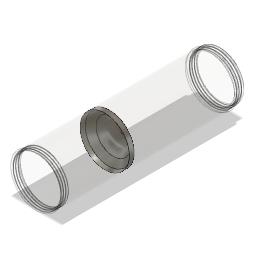
FalconHeavy-SideBoosterBase(No Fin) (Autodesk Fusion 360 design; units mm, degrees)
Autodesk Fusion 360 part; units mm, degrees
sketch "Sketch1" plane through (0, 0, 0) normal (0, 1, 0) x (1, 0, 0)
  line L0 (0, 0) -> (21, 0)
  line L1 (0, 0) -> (20.2, 0)
  line L2 (21, 0) -> (21, 144)
  line L3 (20.2, 0) -> (20.2, 144)
  line L4 (20.2, 144) -> (18.2, 144)
  line L5 (18.2, 144) -> (18.2, 150)
  line L6 (18.2, 150) -> (20.2, 150)
  line L7 (20.2, 150) -> (20.2, 144)
  line L8 (21, 144) -> (20.2, 144)
  line L9 (20.2, 144) -> (20.2, 142)
  spline S0 degree 5 poles (20.2, 142) (20.2, 142.0899) (20.1718, 142.2773) (20.045, 142.5812) (19.7343, 143.0169) (19.2169, 143.5343) (18.7812, 143.845) (18.4773, 143.9718) (18.2899, 144) (18.2, 144) knots 0 0 0 0 0 0 0.2 0.4 0.6 0.8 1 1 1 1 1 1
  line L10 (20.2, 141.8) -> (20.2, 142.2)
  line L11 (18.4, 144) -> (18, 144)
  line L12 (0, 0) -> (0, 150) construction
  line L13 (20.2, 0) -> (20.2, 6)
  line L14 (20.2, 6) -> (0, 6)
  line L15 (20.2, 6) -> (20.2, 7)
  line L16 (20.2, 7) -> (0, 7)
  line L17 (0, 7) -> (0, 6)
  dimension "d1" = 21
  dimension "d2" = 20.2
  dimension "d3" = 144
  dimension "d4" = 144
  dimension "d5" = 2
  dimension "d6" = 6
  dimension "d7" = 2
  dimension "d8" = 2
  dimension "d9" = 150
  dimension "d10" = 6
  dimension "d11" = 1
  constraint coincident L0.start L1.start
  constraint horizontal L0
  constraint parallel L0 L1
  constraint perpendicular L0 L2
  constraint perpendicular L1 L3
  constraint perpendicular L3 L4
  constraint perpendicular L4 L5
  constraint perpendicular L5 L6
  constraint perpendicular L4 L9
  constraint midpoint L9.end L10
  constraint coincident L3 L10.start
  constraint midpoint L4.end L11
  constraint perpendicular L0 L12
  constraint perpendicular L1 L13
  constraint perpendicular L3 L14
  constraint coincident L3 L15.end
  constraint coincident L12 L16.end
  constraint perpendicular L12 L16
  constraint perpendicular L14 L17
  measures "d1" distance of L0.start L0.end
  measures "d2" distance of L0.start L1.end
  measures "d3" distance of L0.end L2.end
  measures "d4" distance of L1.end L3.end
  measures "d5" distance of L3.end L4.end
  measures "d6" distance of L4.end L5.end
  measures "d7" distance of L5.end L6.end
  measures "d8" distance of L3.end L9.end
  measures "d9" distance of L0.start L12.end
  measures "d10" distance of L1.end L13.end
  measures "d11" distance of L13.end L15.end
revolve "Revolve1" add sketch "Sketch1" angle 360 about axis through (0, 0, 0) along (0, 0, -1) makes body 1
thread "Thread1" "ISO Metric profile 40.0 M40x2 6H" major diameter 40.2565 minor diameter 38.0224 pitch 2 angle 60 modelled right hand crest width 0.25 on face at (19.9384, 3.2403, -2) crest through (19.0112, 0, -7.125) on bodies 1
hole "Hole1" at (0, 0, -6) direction (0, 0, -1) diameter 40.4 depth 20 tip angle 180 bodies 1
thread "Thread2" "ISO Metric profile 40.0 M40x2 6g" major diameter 39.822 minor diameter 37.5289 pitch 2 angle 60 modelled right hand crest width 0.25 on face at (20.1749, -1.0069, -146) crest through (19.911, 0, -150.125) on bodies 1
sketch "Sketch1 (2)" plane through (0, 0, 0) normal (0, 1, 0) x (1, 0, 0) in component "Component"
  line L0 (55, 0) -> (76, 0)
  line L1 (76, 0) -> (75.2, 0)
  line L2 (55, 3.5) -> (55, 6.5)
  line L3 (55, 5.777) -> (55, 8.777)
  line L4 (55, 5.777) -> (64, 5.777)
  line L5 (64, 5.777) -> (64, 8.777)
  line L6 (64, 8.777) -> (55, 8.777)
  line L7 (55, 8.777) -> (55, 10.5)
  spline S0 degree 5 poles (55, 10.5) (55.5147, 10.4357) (56.5138, 10.3107) (57.9214, 10.1346) (59.6077, 9.9181) (61.3603, 9.6536) (62.728, 9.3613) (63.7176, 9.0035) (64.3959, 8.5431) (64.9339, 7.9498) (65.5769, 7.2041) (66.5469, 6.3024) (67.9719, 5.261) (69.7789, 4.1244) (71.7331, 2.9573) (73.5241, 1.8315) (74.5715, 1.0174) (75.027, 0.4784) (75.1693, 0.1537) (75.2, 0) knots 0 0 0 0 0 0 0.066667 0.133333 0.2 0.266667 0.333333 0.4 0.466667 0.533333 0.6 0.666667 0.733333 0.8 0.866667 0.933333 1 1 1 1 1 1
  line L8 (75, 1) -> (75.4, -1)
  line L9 (51, 11) -> (59, 10)
  line L10 (67, 6) -> (67, 7)
  line L11 (64, 8.777) -> (64, 9.777)
  line L12 (55, 10.5) -> (55, 11.5)
  spline S1 degree 5 poles (76, 0) (76.0001, 0.2171) (75.9128, 0.6526) (75.5198, 1.3097) (74.5092, 2.2004) (72.6646, 3.3634) (70.5384, 4.5956) (68.4686, 5.8732) (66.7355, 7.142) (65.6173, 8.2072) (65.0146, 8.9717) (64.5358, 9.5112) (63.7817, 9.9344) (62.6942, 10.2954) (61.2795, 10.6184) (59.5328, 10.9227) (57.8776, 11.1574) (56.4937, 11.33) (55.5084, 11.4436) (55, 11.5) knots 0 0 0 0 0 0 0.066667 0.133333 0.2 0.266667 0.333333 0.4 0.466667 0.533333 0.6 0.666667 0.733333 0.8 0.866667 0.933333 1 1 1 1 1 1
  line L13 (75.9996, -1.2974) -> (76.0004, 1.2974)
  line L14 (69.5, 5) -> (64.5, 9)
  line L15 (65.5, 9) -> (62.5, 10.5541)
  line L16 (73.307, 1.9259) -> (76, -4.5)
  line L17 (76, -4.5) -> (76, 0)
  line L18 (73.9361, 0.4248) -> (69.146, 4.534)
  line L19 (75.2, 3.2456) -> (75.2, -3.8) construction
  line L20 (75.2, 1.5091) -> (75.2, -2.5911)
  point P0 (67, 6)
  dimension "d17" = 21
  dimension "d18" = 0.8
  dimension "d24" = 3
  dimension "d25" = 9
  dimension "d26" = 3
  dimension "d27" = 9
  dimension "d28" = 1
  dimension "d29" = 1
  dimension "d30" = 1
  constraint horizontal L0
  constraint parallel L0 L1
  constraint vertical L2
  constraint coincident L2 L3.start
  constraint parallel L2 L3
  constraint perpendicular L3 L4
  constraint perpendicular L4 L5
  constraint perpendicular L6 L7
  constraint midpoint L1.end L8
  constraint midpoint L7.end L9
  constraint coincident P0 L10.start
  constraint vertical L10
  constraint coincident L5.end L6.start
  constraint perpendicular L6 L11
  constraint parallel L7 L12
  constraint midpoint L0.end L13
  constraint midpoint L10.end L14
  constraint midpoint L11.end L15
  constraint coincident S0 L16.start
  constraint coincident L16 L18.start
  constraint coincident S0 L18.end
  constraint vertical L19
  constraint coincident S1 L20.start
  constraint coincident L19 L20.start
  constraint coincident L19 L20.end
  constraint coincident L16 L20.end
  measures "d17" distance of L0.start L0.end
  measures "d18" distance of L0.end L1.end
  measures "d24" distance of L3.start L3.end
  measures "d25" distance of L3.start L4.end
  measures "d26" distance of L4.end L5.end
  measures "d27" distance of L3.end L5.end
  measures "d28" distance of P0 L10.end
  measures "d29" distance of L5.end L11.end
  measures "d30" distance of L7.end L12.end
revolve "Revolve3" add sketch "Sketch1 (2)" angle 360 about axis through (55, 0, -3.5) along (0, 0, -1) separate body contours L0 L16 L20 | L0 S0 L16 | S0 L10 S1 L20 | S0 L16 L18 | S0 L10 L11 S1 | S0 L11 L12 S1 makes body 2 in component "Component"
revolve "Revolve2" add sketch "Sketch1 (2)" angle 360 about axis through (55, 0, -3.5) along (0, 0, -1) separate body contours L0 L1 S1 L20 | L0 L16 L20 | L0 S0 L16 | S0 L10 S1 L20 | L0 L1 L13 L16 L17 L20 | S0 L16 L18 | S0 L10 L11 S1 | S0 L11 L12 S1 makes body 3 in component "Component"
revolve "Revolve1'" add sketch "Sketch1 (2)" angle 360 about axis through (55, 0, -5.777) along (0, 0, -1) separate body contours L0 L1 S1 L20 | S0 L10 S1 L20 | S0 L10 L11 S1 | S0 L11 L12 S1 makes body 4 in component "Component"
move_body "Move1" bodies 4 to x (1, 0, 0) y (0, 1, 0) z (0, 0, 1) at (-55, 0, 10.5) in component "Component"
move_body "Move2" bodies 4 to x (1, 0, 0) y (0, 1, 0) z (0, 0, 1) at (0, 0, -70) in component "Component"
move_body "Move3" bodies 4 to x (1, 0, 0) y (0, 1, 0) z (0, 0, 1) at (0, 0, -2) in component "Component"
move_body "Move4" bodies 4 to x (1, 0, 0) y (0, 1, 0) z (0, 0, 1) at (0, 0, 3) in component "Component"
fillet "Fillet1" radius 10 1 edges at (-18.833, -7.3046, -58.5) on bodies 4 in component "Component"
move_body "Move5" bodies 3 to x (1, 0, 0) y (0, 1, 0) z (0, 0, 1) at (-55, 0, -58.5) in component "Component"
move_body "Move6" bodies 3 to x (1, 0, 0) y (0, 1, 0) z (0, 0, 1) at (0, 0, 1) in component "Component"
delete_body "RemoveBody1" bodies 4 in component "Component"
move_body "Move7" bodies 3 to x (1, 0, 0) y (0, 1, 0) z (0, 0, 1) at (0, 0, -1) in component "Component"
move_body "Move8" bodies 2 to x (1, 0, 0) y (0, 1, 0) z (0, 0, 1) at (-55, 0, -58.5) in component "Component"
delete_body "RemoveBody2" bodies 3 in component "Component"
component "Component" placed x (1, 0, 0) y (0, 1, 0) z (0, 0, 1) at (0, 0, 0)
equation "d2 = 21 mm - Wall_Thickness"
equation "d14 = 42 mm - 2 * Wall_Thickness"
equation "Wall_Thickness = 0.8 mm"
equation "d18 = Wall_Thickness"
